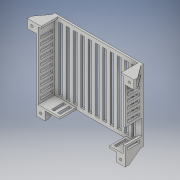
# Autodesk Inventor part: cage
Saved by Autodesk Inventor 2019 (Build 230136000, 136)
## iProperties
Created: 2021-05-18
Part Number: cage
Material: Generisch
Document SubType Name: Modeling
Designer: Michael Hohenstein
Density: 1 g/cm^3
Appearance: Vorgabe
Author: Michael Hohenstein
Autodesk Inventor part; units mm, degrees
ref_plane "YZ Plane" through (0, 0, 0) normal (1, 0, 0) x (0, 1, 0)
ref_plane "XZ Plane" through (0, 0, 0) normal (0, 1, 0) x (-1, 0, 0)
ref_plane "XY Plane" through (0, 0, 0) normal (0, 0, 1) x (1, 0, 0)
sketch "Skizze1" plane through (0, 0, 0) normal (0, 0, 1) x (1, 0, 0)
  line L0 (-45.5, 36.5) -> (45.5, 36.5)
  line L1 (45.5, 36.5) -> (45.5, -36.5)
  line L2 (45.5, -36.5) -> (-45.5, -36.5)
  line L3 (-45.5, -36.5) -> (-45.5, 36.5)
  line L4 (43.5, 34.5) -> (-43.5, 34.5)
  line L5 (-43.5, 34.5) -> (-43.5, -34.5)
  line L6 (-43.5, -34.5) -> (43.5, -34.5)
  line L7 (43.5, -34.5) -> (43.5, 34.5)
  line L8 (-39.5, 32.5) -> (-35.5, 32.5)
  line L9 (-35.5, 32.5) -> (-35.5, -32.5)
  line L10 (-35.5, -32.5) -> (-39.5, -32.5)
  line L11 (-39.5, -32.5) -> (-39.5, 32.5)
  line L12 (-28, 32.5) -> (-28, -32.5)
  line L13 (-32, 32.5) -> (-28, 32.5)
  line L14 (-32, -32.5) -> (-32, 32.5)
  line L15 (-28, -32.5) -> (-32, -32.5)
  line L16 (-20.5, 32.5) -> (-20.5, -32.5)
  line L17 (-24.5, 32.5) -> (-20.5, 32.5)
  line L18 (-24.5, -32.5) -> (-24.5, 32.5)
  line L19 (-20.5, -32.5) -> (-24.5, -32.5)
  line L20 (-13, 32.5) -> (-13, -32.5)
  line L21 (-17, 32.5) -> (-13, 32.5)
  line L22 (-17, -32.5) -> (-17, 32.5)
  line L23 (-13, -32.5) -> (-17, -32.5)
  line L24 (-5.5, 32.5) -> (-5.5, -32.5)
  line L25 (-9.5, 32.5) -> (-5.5, 32.5)
  line L26 (-9.5, -32.5) -> (-9.5, 32.5)
  line L27 (-5.5, -32.5) -> (-9.5, -32.5)
  line L28 (2, 32.5) -> (2, -32.5)
  line L29 (-2, 32.5) -> (2, 32.5)
  line L30 (-2, -32.5) -> (-2, 32.5)
  line L31 (2, -32.5) -> (-2, -32.5)
  line L32 (9.5, 32.5) -> (9.5, -32.5)
  line L33 (5.5, 32.5) -> (9.5, 32.5)
  line L34 (5.5, -32.5) -> (5.5, 32.5)
  line L35 (9.5, -32.5) -> (5.5, -32.5)
  line L36 (17, 32.5) -> (17, -32.5)
  line L37 (13, 32.5) -> (17, 32.5)
  line L38 (13, -32.5) -> (13, 32.5)
  line L39 (17, -32.5) -> (13, -32.5)
  line L40 (24.5, 32.5) -> (24.5, -32.5)
  line L41 (20.5, 32.5) -> (24.5, 32.5)
  line L42 (20.5, -32.5) -> (20.5, 32.5)
  line L43 (24.5, -32.5) -> (20.5, -32.5)
  line L44 (32, 32.5) -> (32, -32.5)
  line L45 (28, 32.5) -> (32, 32.5)
  line L46 (28, -32.5) -> (28, 32.5)
  line L47 (32, -32.5) -> (28, -32.5)
  line L48 (39.5, 32.5) -> (39.5, -32.5)
  line L49 (35.5, 32.5) -> (39.5, 32.5)
  line L50 (35.5, -32.5) -> (35.5, 32.5)
  line L51 (39.5, -32.5) -> (35.5, -32.5)
  point P0 (0, 0)
  point P1 (0, 36.5)
  point P2 (45.5, 0)
  point P3 (-35.5, 0)
  point P4 (-28, 0)
  point P5 (-20.5, 0)
  point P6 (-13, 0)
  point P7 (-5.5, 0)
  point P8 (2, 0)
  point P9 (9.5, 0)
  point P10 (17, 0)
  point P11 (24.5, 0)
  point P12 (32, 0)
  point P13 (39.5, 0)
  point P14 (0, 32.5)
  dimension "d0" = 91
  dimension "d1" = 73
  dimension "d2" = 2
  dimension "d4" = 4
  dimension "d5" = 2
  dimension "d8" = 7.5
  constraints: 104 end point, 6 parallel, 4 midpoint, 3 horizontal, 3 perpendicular, 2 horizontal alignment, 2 vertical alignment, 93 other
  measures "d0" distance of L0.start L0.end
  measures "d1" distance of L0.end L1.end
  measures "d2" distance between parallel lines of L0 L4
  measures "d4" distance of L9.end L10.end
  measures "d5" distance between parallel lines of L4 L8
  measures "d8" distance of L8.end L12.start
extrude "Extrusion1" add sketch "Skizze1" along normal blind 2 contours L0 L1 L2 L3 | L7 L6 L5 L4
sketch "Skizze2" plane through (0, 0, 2) normal (0, 0, 1) x (1, 0, 0)
  line L0 (45.5, 36.5) -> (-45.5, 36.5) construction
  line L1 (-45.5, 36.5) -> (45.5, 36.5) construction
  line L2 (45.5, 36.5) -> (45.5, -36.5) construction
  line L3 (45.5, -36.5) -> (-45.5, -36.5) construction
  line L4 (-45.5, -36.5) -> (-45.5, 36.5) construction
  line L5 (-43.5, 34.5) -> (43.5, 34.5) construction
  line L6 (43.5, 34.5) -> (43.5, -34.5) construction
  line L7 (43.5, -34.5) -> (-43.5, -34.5) construction
  line L8 (-43.5, -34.5) -> (-43.5, 34.5) construction
  line L9 (-45.5, 36.5) -> (-43.5, 36.5)
  line L10 (-43.5, 36.5) -> (-43.5, -36.5)
  line L11 (-43.5, -36.5) -> (-45.5, -36.5)
  line L12 (-45.5, -36.5) -> (-45.5, 36.5)
  line L13 (-45.5, 36.5) -> (-40.5, 36.5)
  line L14 (-40.5, 36.5) -> (-40.5, 34.5)
  line L15 (-40.5, 34.5) -> (-45.5, 34.5)
  line L16 (-45.5, 34.5) -> (-45.5, 36.5)
  line L17 (-45.5, -36.5) -> (-21.5, -36.5)
  line L18 (-21.5, -36.5) -> (-21.5, -34.5)
  line L19 (-21.5, -34.5) -> (-45.5, -34.5)
  line L20 (-45.5, -34.5) -> (-45.5, -36.5)
  line L21 (45.5, -36.5) -> (43.5, -36.5)
  line L22 (43.5, -36.5) -> (43.5, -26.5)
  line L23 (43.5, -26.5) -> (45.5, -26.5)
  line L24 (45.5, -26.5) -> (45.5, -36.5)
  line L25 (45.5, -36.5) -> (29.5, -36.5)
  line L26 (29.5, -36.5) -> (29.5, -34.5)
  line L27 (29.5, -34.5) -> (45.5, -34.5)
  line L28 (45.5, -34.5) -> (45.5, -36.5)
  line L29 (45.5, 36.5) -> (43.5, 36.5)
  line L30 (43.5, 36.5) -> (43.5, -10.5)
  line L31 (43.5, -10.5) -> (45.5, -10.5)
  line L32 (45.5, -10.5) -> (45.5, 36.5)
  line L33 (45.5, 36.5) -> (41.5, 36.5)
  line L34 (41.5, 36.5) -> (41.5, 34.5)
  line L35 (41.5, 34.5) -> (45.5, 34.5)
  line L36 (45.5, 34.5) -> (45.5, 36.5)
  point P0 (0, 0)
  dimension "d15" = 2
  dimension "d16" = 3
  dimension "d17" = 22
  dimension "d18" = 14
  dimension "d19" = 8
  dimension "d20" = 2
  dimension "d21" = 45
  constraints: 72 end point, 18 parallel, 9 perpendicular, 8 horizontal, 7 point on line, 1 vertical alignment, 3 other
  measures "d15" distance between parallel lines of L4 L8
  measures "d16" distance between parallel lines of L14 L10
  measures "d17" distance between parallel lines of L18 L10
  measures "d18" distance from line of L26.end L22
  measures "d19" distance between parallel lines of L27 L23
  measures "d20" distance between parallel lines of L30 L34
  measures "d21" distance from line of L35.end L31
extrude "Extrusion2" add sketch "Skizze2" along normal blind 17
sketch "Skizze3" plane through (-45.5, -36.5, 0) normal (-1, 0, 0) x (0, 0, 1)
  line L0 (2, 71) -> (19, 71) construction
  line L1 (2, 2) -> (19, 2) construction
  line L2 (19, 71) -> (2, 71) construction
  line L3 (2, 71) -> (2, 2) construction
  line L4 (2, 2) -> (19, 2) construction
  line L5 (19, 2) -> (19, 71) construction
  line L6 (16.5, 62) -> (4.5, 62)
  line L7 (4.5, 62) -> (4.5, 59)
  line L8 (4.5, 59) -> (16.5, 59)
  line L9 (16.5, 59) -> (16.5, 62)
  line L10 (16.5, 56) -> (4.5, 56)
  line L11 (4.5, 56) -> (4.5, 53)
  line L12 (4.5, 53) -> (16.5, 53)
  line L13 (16.5, 53) -> (16.5, 56)
  line L14 (16.5, 50) -> (4.5, 50)
  line L15 (4.5, 50) -> (4.5, 47)
  line L16 (4.5, 47) -> (16.5, 47)
  line L17 (16.5, 47) -> (16.5, 50)
  line L18 (16.5, 44) -> (4.5, 44)
  line L19 (4.5, 44) -> (4.5, 41)
  line L20 (4.5, 41) -> (16.5, 41)
  line L21 (16.5, 41) -> (16.5, 44)
  line L22 (16.5, 38) -> (4.5, 38)
  line L23 (4.5, 38) -> (4.5, 35)
  line L24 (4.5, 35) -> (16.5, 35)
  line L25 (16.5, 35) -> (16.5, 38)
  line L26 (16.5, 32) -> (4.5, 32)
  line L27 (4.5, 32) -> (4.5, 29)
  line L28 (4.5, 29) -> (16.5, 29)
  line L29 (16.5, 29) -> (16.5, 32)
  line L30 (16.5, 26) -> (4.5, 26)
  line L31 (4.5, 26) -> (4.5, 23)
  line L32 (4.5, 23) -> (16.5, 23)
  line L33 (16.5, 23) -> (16.5, 26)
  line L34 (16.5, 20) -> (4.5, 20)
  line L35 (4.5, 20) -> (4.5, 17)
  line L36 (4.5, 17) -> (16.5, 17)
  line L37 (16.5, 17) -> (16.5, 20)
  line L38 (16.5, 14) -> (4.5, 14)
  line L39 (4.5, 14) -> (4.5, 11)
  line L40 (4.5, 11) -> (16.5, 11)
  line L41 (16.5, 11) -> (16.5, 14)
  line L42 (16.5, 8) -> (4.5, 8)
  line L43 (4.5, 8) -> (4.5, 5)
  line L44 (4.5, 5) -> (16.5, 5)
  line L45 (16.5, 5) -> (16.5, 8)
  line L46 (0, 0) -> (0, 73) projected
  point P0 (0, 36.5)
  point P1 (10.5, 62)
  point P2 (10.5, 71)
  point P3 (10.5, 56)
  point P4 (10.5, 50)
  point P5 (10.5, 44)
  point P6 (10.5, 38)
  point P7 (10.5, 32)
  point P8 (10.5, 26)
  point P9 (10.5, 20)
  point P10 (10.5, 14)
  point P11 (10.5, 8)
  point P12 (0, 36.5)
  point P13 (4.5, 36.5)
  point P14 (0, 36.5)
  dimension "d24" = 3
  dimension "d25" = 2.5
  dimension "d28" = 6
  constraints: 88 end point, 5 midpoint, 4 parallel, 2 horizontal, 2 perpendicular, 1 horizontal alignment, 1 vertical, 1 vertical alignment, 81 other
  measures "d24" distance of L6.end L7.end
  measures "d25" distance between parallel lines of L3 L7
  measures "d28" distance of L6.start L10.start
extrude "Extrusion3" cut sketch "Skizze3" against normal up to surface (91 mm away)
sketch "Skizze4" plane through (-45.5, -36.5, 0) normal (0, -1, 0) x (1, 0, 0)
  line L0 (5, 2) -> (5, 19) construction
  line L1 (89, 2) -> (89, 19) construction
  line L2 (5, 19) -> (89, 19) construction
  line L3 (89, 19) -> (89, 2) construction
  line L4 (89, 2) -> (5, 2) construction
  line L5 (5, 2) -> (5, 19) construction
  line L6 (13, 16.5) -> (16, 16.5)
  line L7 (16, 16.5) -> (16, 4.5)
  line L8 (16, 4.5) -> (13, 4.5)
  line L9 (13, 4.5) -> (13, 16.5)
  line L10 (19, 16.5) -> (22, 16.5)
  line L11 (22, 16.5) -> (22, 4.5)
  line L12 (22, 4.5) -> (19, 4.5)
  line L13 (19, 4.5) -> (19, 16.5)
  line L14 (24, 2) -> (24, 19) construction
  line L15 (5, 2) -> (24, 2) construction
  line L16 (24, 2) -> (24, 19) construction
  line L17 (24, 19) -> (5, 19) construction
  line L18 (5, 19) -> (5, 2) construction
  line L19 (77, 16.5) -> (80, 16.5)
  line L20 (80, 16.5) -> (80, 4.5)
  line L21 (80, 4.5) -> (77, 4.5)
  line L22 (77, 4.5) -> (77, 16.5)
  line L23 (24, 2) -> (75, 2) construction
  line L24 (75, 2) -> (89, 2) construction
  line L25 (89, 2) -> (89, 19) construction
  line L26 (89, 19) -> (75, 19) construction
  line L27 (75, 19) -> (75, 2) construction
  point P0 (45.5, 0)
  point P1 (13, 10.5)
  point P2 (5, 10.5)
  point P3 (19, 10.5)
  point P4 (14.5, 19)
  point P5 (77, 10.5)
  point P6 (19, 10.5)
  point P7 (82, 19)
  point P8 (14.5, 16.5)
  point P9 (19, 10.5)
  dimension "d35" = 3
  dimension "d36" = 2.5
  dimension "d39" = 6
  dimension "d91" = 2
  constraints: 48 end point, 10 parallel, 7 midpoint, 6 horizontal, 5 perpendicular, 3 horizontal alignment, 2 equal length, 1 vertical alignment, 9 other
  measures "d35" distance of L7.end L8.end
  measures "d36" distance between parallel lines of L2 L6
  measures "d39" distance of L6.start L10.start
  measures "d91" distance between parallel lines of L27 L22
extrude "Extrusion4" cut sketch "Skizze4" against normal up to surface (2 mm away)
sketch "Skizze5" plane through (0, 0, 19) normal (0, 0, 1) x (1, 0, 0)
  line L0 (-45.5, -36.5) -> (-45.5, 36.5) projected
  line L1 (-45.5, -36.5) -> (-36.5, -36.5)
  line L2 (-36.5, -36.5) -> (-36.5, -45.5)
  line L3 (-36.5, -45.5) -> (-45.5, -45.5)
  line L4 (-45.5, -45.5) -> (-45.5, -36.5)
  line L5 (45.5, -36.5) -> (-45.5, -36.5) projected
  line L6 (45.5, -36.5) -> (36.5, -36.5)
  line L7 (36.5, -36.5) -> (36.5, -45.5)
  line L8 (36.5, -45.5) -> (45.5, -45.5)
  line L9 (45.5, -45.5) -> (45.5, -36.5)
  line L10 (-45.5, 36.5) -> (45.5, 36.5) projected
  line L11 (45.5, 36.5) -> (54.5, 36.5)
  line L12 (54.5, 36.5) -> (54.5, 27.5)
  line L13 (54.5, 27.5) -> (45.5, 27.5)
  line L14 (45.5, 27.5) -> (45.5, 36.5)
  line L15 (-45.5, 36.5) -> (-54.5, 36.5)
  line L16 (-54.5, 36.5) -> (-54.5, 27.5)
  line L17 (-54.5, 27.5) -> (-45.5, 27.5)
  line L18 (-45.5, 27.5) -> (-45.5, 36.5)
  circle A0 centre (-50, 32) radius 1.25
  circle A1 centre (50, 32) radius 1.25
  circle A2 centre (41, -41) radius 1.25
  circle A3 centre (-41, -41) radius 1.25
  point P0 (0, 0)
  point P1 (-50, 36.5)
  point P2 (50, 36.5)
  point P3 (41, -45.5)
  point P4 (-41, -45.5)
  point P5 (-54.5, 32)
  point P6 (54.5, 32)
  point P7 (36.5, -41)
  point P8 (-36.5, -41)
  dimension "d53" = 2.5
  dimension "d54" = 9
  constraints: 32 end point, 8 midpoint, 8 parallel, 7 equal length, 4 centre point, 4 horizontal, 4 horizontal alignment, 4 perpendicular, 4 vertical alignment, 3 equal radius
  measures "d53" diameter of A0
  measures "d54" distance of L15.end L16.end
extrude "Extrusion5" add sketch "Skizze5" against normal blind 3
sketch "Skizze6" plane through (0, 0, 16) normal (0, 0, -1) x (-1, 0, 0)
  line L0 (-45.5, 36.5) -> (-45.5, 27.5) projected
  line L1 (-54.5, 36.5) -> (-54.5, 27.5) projected
  line L2 (-45.5, 36.5) -> (-54.5, 36.5)
  line L3 (-54.5, 36.5) -> (-54.5, 35.5)
  line L4 (-54.5, 35.5) -> (-45.5, 35.5)
  line L5 (-45.5, 35.5) -> (-45.5, 36.5)
  line L6 (-45.5, -10.5) -> (-45.5, 27.5) projected
  line L7 (-45.5, 27.5) -> (-54.5, 27.5)
  line L8 (-54.5, 27.5) -> (-54.5, 28.5)
  line L9 (-54.5, 28.5) -> (-45.5, 28.5)
  line L10 (-45.5, 28.5) -> (-45.5, 27.5)
  line L11 (45.5, -36.5) -> (45.5, 36.5) projected
  line L12 (54.5, 36.5) -> (54.5, 27.5) projected
  line L13 (45.5, 36.5) -> (54.5, 36.5)
  line L14 (54.5, 36.5) -> (54.5, 35.5)
  line L15 (54.5, 35.5) -> (45.5, 35.5)
  line L16 (45.5, 35.5) -> (45.5, 36.5)
  line L17 (54.5, 27.5) -> (45.5, 27.5) projected
  line L18 (45.5, 27.5) -> (54.5, 27.5)
  line L19 (54.5, 27.5) -> (54.5, 28.5)
  line L20 (54.5, 28.5) -> (45.5, 28.5)
  line L21 (45.5, 28.5) -> (45.5, 27.5)
  line L22 (36.5, -45.5) -> (36.5, -36.5) projected
  line L23 (36.5, -45.5) -> (45.5, -45.5) projected
  line L24 (36.5, -36.5) -> (37.5, -36.5)
  line L25 (37.5, -36.5) -> (37.5, -45.5)
  line L26 (37.5, -45.5) -> (36.5, -45.5)
  line L27 (36.5, -45.5) -> (36.5, -36.5)
  line L28 (45.5, -36.5) -> (44.5, -36.5)
  line L29 (44.5, -36.5) -> (44.5, -45.5)
  line L30 (44.5, -45.5) -> (45.5, -45.5)
  line L31 (45.5, -45.5) -> (45.5, -36.5)
  line L32 (-45.5, -36.5) -> (-36.5, -36.5) projected
  line L33 (-45.5, -45.5) -> (-36.5, -45.5) projected
  line L34 (-45.5, -36.5) -> (-44.5, -36.5)
  line L35 (-44.5, -36.5) -> (-44.5, -45.5)
  line L36 (-44.5, -45.5) -> (-45.5, -45.5)
  line L37 (-45.5, -45.5) -> (-45.5, -36.5)
  line L38 (-36.5, -45.5) -> (-36.5, -36.5) projected
  line L39 (-36.5, -36.5) -> (-37.5, -36.5)
  line L40 (-37.5, -36.5) -> (-37.5, -45.5)
  line L41 (-37.5, -45.5) -> (-36.5, -45.5)
  line L42 (-36.5, -45.5) -> (-36.5, -36.5)
  point P0 (0, 0)
  dimension "d57" = 1
  dimension "d58" = 1
  dimension "d59" = 1
  dimension "d60" = 1
  dimension "d61" = 1
  dimension "d62" = 1
  dimension "d63" = 1
  dimension "d64" = 1
  constraints: 64 end point, 16 parallel, 8 horizontal, 8 perpendicular, 8 point on line
  measures "d57" distance between parallel lines of L2 L4
  measures "d58" distance between parallel lines of L7 L9
  measures "d59" distance between parallel lines of L13 L15
  measures "d60" distance between parallel lines of L17 L20
  measures "d61" distance between parallel lines of L22 L25
  measures "d62" distance between parallel lines of L31 L29
  measures "d63" distance between parallel lines of L35 L37
  measures "d64" distance between parallel lines of L38 L40
extrude "Extrusion6" add sketch "Skizze6" along normal blind 1 contours L0 L4 L1 L2 | L0 L7 L1 L9 | L11 L20 L12 L17 | L31 L23 L29 L28 | L23 L22 L24 L25 | L11 L13 L12 L15 | L32 L35 L33 L37 | L32 L38 L33 L40
chamfer "Fase1" distance 12 distance2 9 1 edges at (45.5, 36, 15) measured on face at (45.5, 32.5, 6.5)
chamfer "Fase2" distance 12 distance2 9 1 edges at (45.5, 28, 15) measured on face at (45.5, 10.1667, 2.1667)
chamfer "Fase3" distance 12 distance2 9 1 edges at (45, -36.5, 15) measured on face at (9.8333, -36.5, 0.6667)
chamfer "Fase4" distance 12 distance2 9 1 edges at (37, -36.5, 15) measured on face at (9.8333, -36.5, 0.6667)
chamfer "Fase5" distance 12 distance2 9 1 edges at (-37, -36.5, 15) measured on face at (9.8333, -36.5, 0.6667)
chamfer "Fase6" distance 12 distance2 9 1 edges at (-45, -36.5, 15) measured on face at (9.8333, -36.5, 0.6667)
chamfer "Fase7" distance 12 distance2 9 1 edges at (-45.5, 36, 15) measured on face at (-45.5, -5.5, 1.5)
chamfer "Fase8" distance 12 distance2 9 1 edges at (-45.5, 28, 15) measured on face at (-45.5, -5.5, 1.5)
equation "\"d58\" = d57"
equation "\"d59\" = d57"
equation "\"d60\" = d57"
equation "\"d61\" = d57"
equation "\"d62\" = d57"
equation "\"d63\" = d57"
equation "\"d64\" = d57"
